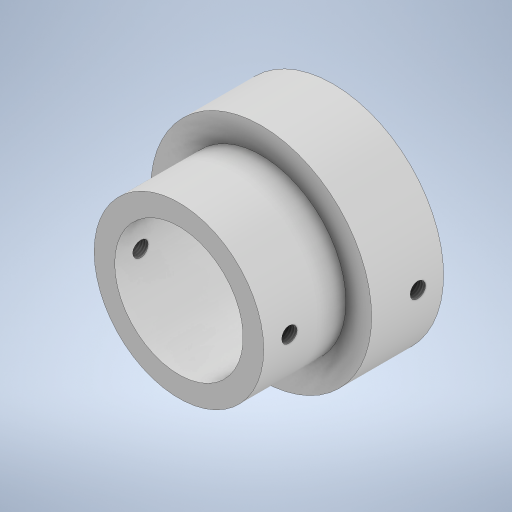
# Autodesk Inventor part: Муфта штурвал, двигатель
Saved by Autodesk Inventor 2023 (Build 270158000, 158)
## iProperties
Created: 2022-05-23
Part Number: Муфта штурвал, двигатель
Material: Типовые
Document SubType Name: Modeling
Designer: User
Density: 1 g/cm^3
Appearance: По умолчанию
Author: User
Autodesk Inventor part; units mm, degrees
ref_plane "YZ Plane" through (0, 0, 0) normal (1, 0, 0) x (0, 1, 0)
ref_plane "XZ Plane" through (0, 0, 0) normal (0, 1, 0) x (-1, 0, 0)
ref_plane "XY Plane" through (0, 0, 0) normal (0, 0, 1) x (1, 0, 0)
sketch "Эскиз1" plane through (0, 0, 0) normal (0, 1, 0) x (-1, 0, 0)
  line L0 (0, 0) -> (12.5, 0)
  line L1 (12.5, 0) -> (16.5, 0)
  line L2 (16.5, 0) -> (16.5, -20)
  line L3 (12.5, 0) -> (12.5, -20)
  line L4 (12.5, -20) -> (16.5, -20)
  line L5 (12.5, -20) -> (0, -20)
  line L6 (0, -20) -> (0, -30)
  line L7 (0, -30) -> (17.5, -30)
  line L8 (17.5, -30) -> (17.5, -20)
  line L9 (17.5, -20) -> (16.5, -20)
  line L10 (17.5, -30) -> (21.5, -30)
  line L11 (21.5, -30) -> (21.5, -16)
  line L12 (21.5, -16) -> (16.5, -16)
  dimension "d0" = 12.5
  dimension "d1" = 4
  dimension "d2" = 20
  dimension "d3" = 10
  dimension "d4" = 17.5
  dimension "d5" = 4
  dimension "d6" = 14
  constraints: 26 end point, 8 perpendicular, 5 point on line, 1 horizontal, 1 vertical
  measures "d0" distance of L0.start L0.end
  measures "d1" distance of L0.end L1.end
  measures "d2" distance of L1.end L2.end
  measures "d3" distance of L5.end L6.end
  measures "d4" distance of L6.end L7.end
  measures "d5" distance of L7.end L10.end
  measures "d6" distance of L10.end L11.end
revolve "Вращение1" add sketch "Эскиз1" angle 360 about axis through (0, 0, -20) along (0, 0, -1) contours L1 L2 L4 L3 | L12 L11 L10 L8 L9 L2
sketch "Эскиз2" plane through (0, 0, 0) normal (1, 0, 0) x (0, 1, 0)
  line L0 (0, 0) -> (0, -5)
  line L1 (-17.5, -30) -> (17.5, -30) projected
  line L2 (0, -30) -> (0, -20)
  line L3 (0, -20) -> (0, -25)
  circle A0 centre (0, -5) radius 1.5
  circle A1 centre (0, -25) radius 1.5
  dimension "d8" = 5
  dimension "d9" = 10
  dimension "d10" = 5
  dimension "d11" = 3
  dimension "d12" = 3
  constraints: 6 end point, 2 centre point, 2 coincident, 2 midpoint, 1 point on line, 1 vertical
  measures "d8" distance of L0.start L0.end
  measures "d9" distance of L2.start L2.end
  measures "d10" distance of L2.end L3.end
  measures "d11" diameter of A0
  measures "d12" diameter of A1
extrude "Выдавливание1" cut sketch "Эскиз2" along normal blind 29.75 and the other way blind 30.75
thread "Резьба1" size "M3x0.5" class "6H" standard "ANSI Metric M Profile" full length
thread "Резьба2" size "M3x0.5" class "6H" standard "ANSI Metric M Profile" full length
